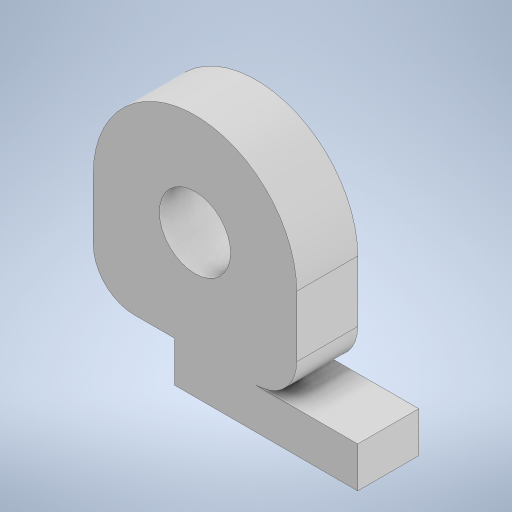
# Autodesk Inventor part: Knuckle Attachment SMALL HOLE
Saved by Autodesk Inventor 2023 (Build 270158000, 158)
## iProperties
Created: 2023-04-04
Part Number: Knuckle Attachment SMALL HOLE
Material: Generic
Document SubType Name: Modeling
Designer: 1senadi
Density: 1 g/cm^3
Appearance: Default
Author: 1senadi
Autodesk Inventor part; units mm, degrees
ref_plane "YZ Plane" through (0, 0, 0) normal (1, 0, 0) x (0, 1, 0)
ref_plane "XZ Plane" through (0, 0, 0) normal (0, 1, 0) x (-1, 0, 0)
ref_plane "XY Plane" through (0, 0, 0) normal (0, 0, 1) x (1, 0, 0)
sketch "Sketch1" plane through (0, 0, 0) normal (0, 1, 0) x (-1, 0, 0)
  line L0 (0, 0) -> (0, -3)
  line L1 (0, -3) -> (10, -3)
  line L2 (10, -3) -> (10, 0)
  line L3 (10, 0) -> (0, 0)
  dimension "d0" = 3
  dimension "d1" = 10
  dimension "d2" = 90
  dimension "d3" = 3
  constraints: 8 end point, 2 perpendicular, 1 vertical
  measures "d0" distance of L0.start L0.end
  measures "d1" distance of L0.end L1.end
  measures "d2" angle of L1 L0
  measures "d3" distance of L1.end L2.end
extrude "Extrusion1" add sketch "Sketch1" along normal blind 12
sketch "Sketch4" plane through (0, 0, -3) normal (0, 0, -1) x (-1, 0, 0)
  line L0 (0, 0) -> (0, 2)
  line L1 (0, 0) -> (0, 12) projected
  line L2 (0, 2) -> (4, 2)
  line L3 (10, 0) -> (10, 12) projected
  line L4 (4, 2) -> (0, 0)
  line L5 (0, 0) -> (10, 0) projected
  line L6 (10, 0) -> (10, 2)
  line L7 (10, 2) -> (6, 2)
  line L8 (6, 2) -> (10, 0)
  line L9 (4, 2) -> (6, 2)
  line L10 (6, 2) -> (6, 0)
  line L11 (4, 2) -> (4, 0)
  line L12 (4, 0) -> (6, 0)
  dimension "d9" = 2
  dimension "d10" = 4
  dimension "d11" = 2
  dimension "d12" = 4
  constraints: 20 end point, 4 perpendicular, 4 point on line, 1 collinear
  measures "d9" distance of L0.start L0.end
  measures "d10" distance of L0.end L2.end
  measures "d11" distance of L3.start L6.end
  measures "d12" distance of L6.end L7.end
extrude "Extrusion3" cut sketch "Sketch4" against normal up to surface (3 mm away) contours L0 L2 L4 | L4 L11 L5 | L7 L3 L8 | L8 L5 L10
sketch "Sketch6" plane through (0, 12, -3) normal (0, 0, -1) x (-1, 0, 0)
  line L0 (0, -10) -> (0, 0) projected
  line L1 (0, -5) -> (10, -5)
  line L2 (10, -10) -> (10, 0) projected
  line L3 (0, 0) -> (10, 0) projected
  line L4 (5, 0) -> (5, -10)
  circle A0 centre (5, -5) radius 1.75
  point P0 (0, -12)
  dimension "d15" = 3.5
  constraints: 4 end point, 4 midpoint, 1 centre point, 1 vertical
  measures "d15" diameter of A0
extrude "Extrusion4" cut sketch "Sketch6" against normal up to surface (3 mm away) contours A0 L4 L1 | L1 L4 A0 | L4 A0 L1 | L1 A0 L4
fillet "Fillet1" radius 2 4 edges at (0, 12, -1.5) (0, 2, -1.5) (-10, 12, -1.5) (-10, 2, -1.5)
sketch "Sketch7" plane through (-8, 12, 0) normal (0, 0, 1) x (1, 0, 0)
  circle A0 centre (3, -5) radius 1.75 projected
  arc A1 (8, -2) -> (6, 0) centre (6, -2) ccw projected
  circle A2 centre (3, -5) radius 5
  line L0 (6, 0) -> (0, 0) projected
  line L1 (2, -12) -> (4, -12) projected
  line L2 (4, -10) -> (6, -10) projected
  arc A3 (6, -10) -> (8, -8) centre (6, -8) ccw projected
  line L3 (8, -8) -> (8, -2) projected
  arc A4 (8, -2) -> (6, 0) centre (6, -2) ccw projected
  line L4 (0, 0) -> (6, 0) projected
  arc A5 (0, 0) -> (-2, -2) centre (0, -2) ccw projected
  line L5 (-2, -8) -> (-2, -2) projected
  arc A6 (-2, -8) -> (0, -10) centre (0, -8) ccw projected
  line L6 (0, -10) -> (2, -10) projected
  circle A7 centre (3, -5) radius 1.75 projected
  line L7 (2, -10) -> (2, -12) projected
  line L8 (4, -12) -> (4, -10) projected
  point P0 (8, -12)
  point P1 (-2, -5)
  point P2 (3, 0)
  point P3 (8, -5)
  point P4 (8, -2)
  constraints: 1 centre point, 1 coincident, 1 tangent
extrude "Extrusion5" cut sketch "Sketch7" against normal up to surface (3 mm away) contours L3 A2 L0 A1 | A2 L5 A5 L0
sketch "Sketch8" plane through (-4, 0, -3) normal (1, 0, 0) x (0, 0, -1)
  line L0 (0, 2) -> (0, 0) projected
  line L1 (-3, 0) -> (-3, 2) projected
  line L2 (0, 0) -> (-3, 0)
  line L3 (-3, 0) -> (-3, 2)
  line L4 (-3, 2) -> (0, 2)
  line L5 (0, 2) -> (0, 0)
  constraints: 8 end point, 2 parallel, 1 horizontal, 1 perpendicular
extrude "Extrusion6" add sketch "Sketch8" along normal blind 7
body "Solid1"
